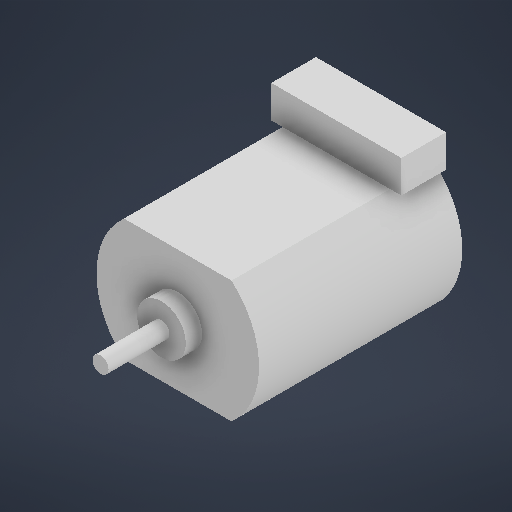
# Autodesk Inventor part: Мотор
Saved by Autodesk Inventor 2026.2 (Build 302298000, 298)
## iProperties
Created: 2026-02-21
Part Number: Мотор
Material: Типовые
Document SubType Name: Modeling
Designer: Leonid
Density: 1 g/cm^3
Appearance: По умолчанию
Author: Leonid
Autodesk Inventor part; units mm, degrees
ref_plane "YZ Plane" through (0, 0, 0) normal (1, 0, 0) x (0, 1, 0)
ref_plane "XZ Plane" through (0, 0, 0) normal (0, 1, 0) x (-1, 0, 0)
ref_plane "XY Plane" through (0, 0, 0) normal (0, 0, 1) x (1, 0, 0)
sketch "Эскиз1" plane through (0, 0, 0) normal (0, 0, 1) x (1, 0, 0)
  line L0 (-10, 7.5) -> (-6.6144, 7.5) construction
  line L1 (10, 7.5) -> (10, -7.5) construction
  line L2 (10, -7.5) -> (6.6144, -7.5) construction
  line L3 (-10, -7.5) -> (-10, 7.5) construction
  line L4 (-10, 7.5) -> (10, -7.5) construction
  line L5 (10, 7.5) -> (-10, -7.5) construction
  arc A0 (-6.6144, 7.5) -> (-6.6144, -7.5) centre (0, 0) ccw
  arc A1 (6.6144, -7.5) -> (6.6144, 7.5) centre (0, 0) ccw
  line L6 (-6.6144, 7.5) -> (6.6144, 7.5)
  line L7 (-6.6144, -7.5) -> (-10, -7.5) construction
  line L8 (6.6144, -7.5) -> (-6.6144, -7.5)
  line L9 (6.6144, 7.5) -> (10, 7.5) construction
  circle A2 centre (0, 0) radius 3
  circle A3 centre (0, 0) radius 1
  point P0 (10, 0)
  point P1 (-10, 0)
  dimension "d0" = 20
  dimension "d1" = 15
  dimension "d4" = 6
  dimension "d7" = 2
  constraints: 20 end point, 10 parallel, 6 point on circle, 4 centre point, 4 midpoint, 3 coincident, 3 horizontal, 3 perpendicular, 1 point on line
  measures "d0" distance of L1.end L3.start
  measures "d1" distance of L1.start L1.end
  measures "d4" diameter of A2
  measures "d7" diameter of A3
extrude "Выдавливание1" add sketch "Эскиз1" against normal blind 25 contours L6 A1 L8 A0 | A2 | A3
extrude "Выдавливание2" add sketch "Эскиз1" along normal blind 2 contours A2 | A3
extrude "Выдавливание3" add sketch "Эскиз1" along normal blind 9.5 contours A3
sketch "Эскиз4" plane through (0, 0, -25) normal (0, 0, -1) x (-1, 0, 0)
  arc A0 (3, -4) -> (-3, -4) centre (0, 0) ccw
  line L0 (-3, -4) -> (3, -4)
  arc A1 (-3, -4) -> (3, -4) centre (0, 0) ccw construction
  circle A2 centre (0, 0) radius 1
  point P0 (0, 5)
  dimension "d10" = 10
  dimension "d13" = 9
  dimension "d14" = 2
  constraints: 5 point on circle, 3 centre point, 2 coincident, 2 end point, 1 horizontal
  measures "d10" diameter of A0
  measures "d13" distance from line of L0 point (0, 5)
  measures "d14" diameter of A2
extrude "Выдавливание4" add sketch "Эскиз4" along normal blind 2.5 contours L0 A0 | A2
extrude "Выдавливание5" add sketch "Эскиз4" along normal blind 3.75 contours A2
sketch "Эскиз5" plane through (-6.6144, 7.5, 0) normal (0, 1, 0) x (1, 0, 0)
  line L0 (13.2288, 0) -> (0, 0) projected
  line L1 (13.2288, 0) -> (13.2288, 25) projected
  line L2 (0, 25) -> (13.2288, 25) projected
  line L3 (0, 0) -> (0, 25) projected
  line L4 (13.2288, 19.5) -> (0, 19.5)
  line L5 (13.2288, 19.5) -> (14.6144, 19.5)
  line L6 (13.2288, 25) -> (14.6144, 25)
  line L7 (16.6144, 25) -> (13.2288, 25) projected
  line L8 (14.6144, 19.5) -> (14.6144, 25)
  line L9 (0, 19.5) -> (-1.3856, 19.5)
  line L10 (0, 25) -> (-1.3856, 25)
  line L11 (0, 25) -> (-3.3856, 25) projected
  line L12 (-1.3856, 19.5) -> (-1.3856, 25)
  point P0 (6.6144, 0)
  dimension "d17" = 5.5
  dimension "d18" = 16
  constraints: 14 end point, 4 point on line, 3 perpendicular, 2 horizontal, 1 collinear
  measures "d17" distance between parallel lines of L4 L2
  measures "d18" distance between parallel lines of L12 L8
extrude "Выдавливание6" add sketch "Эскиз5" along normal blind 4 contours L4 L3 L2 L1 | L1 L6 L8 L5 | L9 L12 L10 L3
